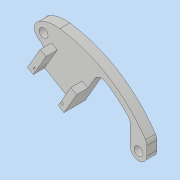
# Autodesk Inventor part: BatteryBalanceConnectorHolder
Saved by Autodesk Inventor 2017 (Build 210142000, 142)
## iProperties
Created: 2019-07-16
Part Number: BatteryBalanceConnectorHolder
Material: Generic
Document SubType Name: Modeling
Designer: techn
Density: 1 g/cm^3
Appearance: Default
Author: techn
Autodesk Inventor part; units mm, degrees
ref_plane "YZ Plane" through (0, 0, 0) normal (1, 0, 0) x (0, 1, 0)
ref_plane "XZ Plane" through (0, 0, 0) normal (0, 1, 0) x (-1, 0, 0)
ref_plane "XY Plane" through (0, 0, 0) normal (0, 0, 1) x (1, 0, 0)
sketch "Sketch1" plane through (0, 0, 0) normal (0, 0, 1) x (1, 0, 0)
  circle A0 centre (0, 0) radius 1.7145
  arc A1 (-1.687, 3.0581) -> (3.0246, -1.7462) centre (0, 0) ccw
  circle A2 centre (36.2951, -20.955) radius 1.7145
  arc A3 (33.5455, -19.3675) -> (39.4701, -20.955) centre (36.2951, -20.955) ccw
  line L0 (0, 0) -> (44.3838, 0) construction
  arc A4 (39.4701, -16.6464) -> (6.2054, 4.5403) centre (0, -41.91) ccw
  line L1 (33.1201, -20.955) -> (33.1201, -12.2644)
  line L2 (39.4701, -20.955) -> (39.4701, -16.6464)
  arc A5 (6.2054, 4.5403) -> (-1.687, 3.0581) centre (4.5073, -8.1706) ccw
  line L3 (0, 0) -> (36.2951, -20.955) construction
  line L4 (3.0246, -1.7462) -> (-1.8014, -10.1051)
  line L5 (-1.8014, -10.1051) -> (12.1007, -18.1315)
  line L6 (12.1007, -18.1315) -> (16.9267, -9.7726)
  line L7 (16.9267, -9.7726) -> (20.993, -2.7297)
  arc A6 (33.1201, -12.2644) -> (20.993, -2.7297) centre (0, -41.91) ccw
  dimension "d0" = 3.429
  dimension "d1" = 6.985
  dimension "d2" = 3.429
  dimension "d3" = 6.35
  dimension "d4" = 30
  dimension "d5" = 41.91
  dimension "d6" = 93.726
  dimension "d7" = 41.91
  dimension "d10" = 16.0528
  dimension "d11" = 9.652
  constraints: 16 end point, 11 point on circle, 7 centre point, 4 coincident, 4 tangent, 3 perpendicular, 3 point on line, 2 vertical, 1 collinear, 1 horizontal, 1 vertical alignment
  measures "d0" diameter of A0
  measures "d1" diameter of A1
  measures "d2" diameter of A2
  measures "d3" diameter of A3
  measures "d5" distance of point (0, 0) A2.centre
  measures "d6" diameter of A4
  measures "d7" distance of A4.centre point (0, 0)
  measures "d10" distance between parallel lines of L4 L6
  measures "d11" distance of L5.end L6.end
extrude "Extrusion1" add sketch "Sketch1" along normal blind 3.81
fillet "Fillet1" radius 3.175 4 edges at (3.0246, -1.7462, 1.905) (20.993, -2.7297, 1.905) (33.1201, -12.2644, 1.905) (39.4701, -16.6464, 1.905)
sketch "Sketch2" plane through (0, 0, 3.81) normal (0, 0, 1) x (1, 0, 0)
  line L0 (-1.8014, -10.1051) -> (12.1007, -18.1315) projected
  line L1 (12.1007, -18.1315) -> (9.901, -16.8615)
  line L2 (14.727, -8.5026) -> (16.9267, -9.7726)
  line L3 (12.1007, -18.1315) -> (19.3978, -5.4927) projected
  line L4 (12.1007, -18.1315) -> (16.9267, -9.7726)
  line L5 (-0.3054, -7.5139) -> (-1.8014, -10.1051) projected
  line L6 (-1.8014, -10.1051) -> (3.0246, -1.7463)
  line L7 (3.0246, -1.7463) -> (5.2243, -3.0163)
  line L8 (0.3983, -11.3751) -> (-1.8014, -10.1051)
  line L9 (11.171, -14.6618) -> (12.0509, -15.1698)
  line L10 (12.0509, -15.1698) -> (11.5429, -16.0497)
  line L11 (11.5429, -16.0497) -> (10.663, -15.5417)
  line L12 (1.6683, -9.1754) -> (0.7884, -8.6674)
  line L13 (0.7884, -8.6674) -> (0.2804, -9.5473)
  line L14 (0.2804, -9.5473) -> (1.1603, -10.0553)
  line L15 (5.2243, -3.0163) -> (1.6683, -9.1754)
  line L16 (1.1603, -10.0553) -> (0.3983, -11.3751)
  line L17 (9.901, -16.8615) -> (10.663, -15.5417)
  line L18 (11.171, -14.6618) -> (14.727, -8.5026)
  point P0 (0, 0)
  dimension "d15" = 9.652
  dimension "d17" = 2.54
  dimension "d18" = 7.112
  dimension "d19" = 7.112
  dimension "d20" = 1.016
  dimension "d21" = 1.016
  constraints: 32 end point, 18 perpendicular, 3 equal length, 3 point on line, 2 parallel, 1 collinear
  measures "d15" distance of L1.end L2.start
  measures "d17" distance of L2.start L2.end
  measures "d18" distance of L2.start L9.start
  measures "d19" distance of L7.end L12.start
  measures "d20" distance of L12.end L13.end
  measures "d21" distance of L13.end L14.end
extrude "Extrusion2" add sketch "Sketch2" along normal blind 4.318
body "Solid1"
